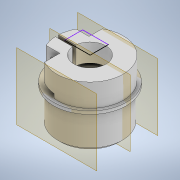
# Autodesk Inventor part: Probe holder
Saved by Autodesk Inventor 2021 (Build 250183000, 183)
## iProperties
Created: 2020-12-21
Part Number: Probe holder
Material: Generic
Document SubType Name: Modeling
Designer: Olivi
Density: 1 g/cm^3
Appearance: Default
Author: Olivi
Autodesk Inventor part; units mm, degrees
ref_plane "YZ Plane" through (0, 0, 0) normal (1, 0, 0) x (0, 1, 0)
ref_plane "XZ Plane" through (0, 0, 0) normal (0, 1, 0) x (-1, 0, 0)
ref_plane "XY Plane" through (0, 0, 0) normal (0, 0, 1) x (1, 0, 0)
sketch "Sketch1" plane through (0, 0, 0) normal (0, 1, 0) x (-1, 0, 0)
  circle A0 centre (0, 0) radius 21.35
  dimension "d0" = 42.7
  constraints: 1 centre point, 1 coincident
  measures "d0" diameter of A0
extrude "Extrusion1" add sketch "Sketch1" along normal blind 23
sketch "Sketch2" plane through (0, 23, 0) normal (0, 1, 0) x (1, 0, 0)
  circle A0 centre (0, 0) radius 24
  dimension "d3" = 48
  constraints: 1 centre point, 1 coincident
  measures "d3" diameter of A0
extrude "Extrusion2" add sketch "Sketch2" along normal blind 2
sketch "Sketch3" plane through (0, 25, 0) normal (0, 1, 0) x (1, 0, 0)
  circle A0 centre (0, 0) radius 24 projected
  circle A1 centre (0, 0) radius 21.9
  dimension "d6" = 43.8
  constraints: 1 centre point, 1 coincident
  measures "d6" diameter of A1
extrude "Extrusion3" add sketch "Sketch3" along normal blind 15 contours A1
sketch "Sketch5" plane through (0, 40, 0) normal (0, 1, 0) x (1, 0, 0)
  line L0 (0, 0) -> (-16.9119, 0)
  line L1 (-16.9119, 0) -> (-16.9119, 11.9609)
  line L2 (-16.9119, 11.9609) -> (0, 11.9609)
  line L3 (0, 11.9609) -> (0, 0)
  constraints: 8 end point, 2 parallel, 1 horizontal, 1 perpendicular
sketch "Sketch8" plane through (0, 40, 0) normal (0, 1, 0) x (1, 0, 0)
  circle A0 centre (0, 0) radius 10.5
  dimension "d18" = 21
  constraints: 1 centre point, 1 coincident
  measures "d18" diameter of A0
extrude "Extrusion5" cut sketch "Sketch8" against normal through all
sketch "Sketch9" plane through (0, 40, 0) normal (0, 1, 0) x (1, 0, 0)
  arc A0 (-20.347, 8.1) -> (20.347, 8.1) centre (0, 0) ccw projected
  line L0 (-21.9, 0) -> (-10.9, 0)
  line L1 (-10.9, 0) -> (-10.9, -21.2976)
  line L2 (-10.9, -21.2976) -> (-22.7633, -21.2976)
  line L3 (-22.7633, -21.2976) -> (-22.7633, 0)
  line L4 (-22.7633, 0) -> (-21.9, 0)
  line L5 (-22.7633, 0) -> (-22.7633, 1)
  line L6 (-22.7633, 1) -> (-8.5921, 1)
  line L7 (-8.5921, 1) -> (-8.5921, -0.9996)
  line L8 (-8.5921, -0.9996) -> (-22.7633, -0.9996)
  line L9 (-10.9, -0.9996) -> (-10.9, -8.9996)
  line L10 (-10.9, -8.9996) -> (-22.7633, -8.9996)
  point P0 (-19.9654, -8.9996)
  point P1 (-10.9, -18.9947)
  dimension "d21" = 11
  dimension "d22" = 1
  dimension "d23" = 8
  constraints: 22 end point, 7 point on line, 6 perpendicular, 1 collinear, 1 horizontal, 1 point on circle, 1 vertical
  measures "d21" distance of L0.start L0.end
  measures "d22" distance of L3.end L5.end
  measures "d23" distance of L9.start L9.end
extrude "Extrusion6" cut sketch "Sketch9" against normal blind 15 contours L6 L7 L8 L1 L0 A0 | A0 L4 L5 L6 | L0 L1 L8 A0 | A0 L8 L3 L4 | L10 L1 A0
sketch "Sketch10" plane through (-19.9654, 40, 8.9996) normal (0, 0, 1) x (1, 0, 0)
  circle A0 centre (4.7692, -6.5146) radius 2.55
  point P0 (19.9654, -40)
  dimension "d26" = 5.1
  constraints: 1 centre point
  measures "d26" diameter of A0
hole "Hole1" at (-15.1962, 33.4854, 8.9996) direction (0, 0, -1) diameter 4.134 end through all thread size "M5x0.8" class "6H" standard "ISO Metric profile"
chamfer "Chamfer1" distance 2 angle 45 1 edges at (21.35, 0, 0)
ref_plane "Work Plane4" through (-21.8772, 40, -0.0002) normal (0, 0, 1) x (1, 0, 0)
ref_plane "Work Plane5" through (-21.8772, 40, 21.9998) normal (0, 0, 1) x (1, 0, 0)
sketch "Sketch11" plane through (-21.8772, 40, 21.9998) normal (0, 0, 1) x (1, 0, 0)
  line L0 (0, -15) -> (1.9118, -15) projected
  line L1 (0, -15) -> (0, -12)
  line L2 (0, 0) -> (0, -15) projected
  line L3 (0, -12) -> (20, -12)
  line L4 (20, -12) -> (20, -15)
  line L5 (20, -15) -> (0, -15)
  line L6 (45.8772, -15) -> (-2.1228, -15) projected
  point P0 (21.8772, -40)
  point P1 (10.9772, -15)
  dimension "d39" = 3
  dimension "d42" = 20
  constraints: 8 end point, 2 perpendicular, 1 collinear, 1 point on line
  measures "d39" distance of L0.start L1.end
  measures "d42" distance of L1.end L3.end
extrude "Extrusion7" cut sketch "Sketch11" against normal through all
ref_plane "Work Plane6" through (-21.8772, 40, -18.2502) normal (0, 0, 1) x (1, 0, 0)
sketch "Sketch13" plane through (-21.8772, 40, -18.2502) normal (0, 0, 1) x (1, 0, 0)
  line L0 (11.4249, 0) -> (11.4249, -12) projected
  line L1 (10.9772, 0) -> (11.4249, -12)
  line L2 (0, -12) -> (0, 0) projected
  line L3 (11.4249, -12) -> (0, -12)
  line L4 (0, -12) -> (0, 0)
  line L5 (0, 0) -> (11.201, 0)
  line L6 (1.9118, 0) -> (10.9772, 0) projected
  line L7 (11.201, 0) -> (11.201, -12)
  line L8 (11.4248, -12) -> (0, -12) projected
  point P0 (21.8772, -40)
  point P1 (11.201, -6)
  constraints: 10 end point, 2 collinear, 2 perpendicular, 1 point on line
extrude "Extrusion9" cut sketch "Sketch13" along normal mid plane 16 contours L1 L7 L3 L2 L5
body "Solid1"
